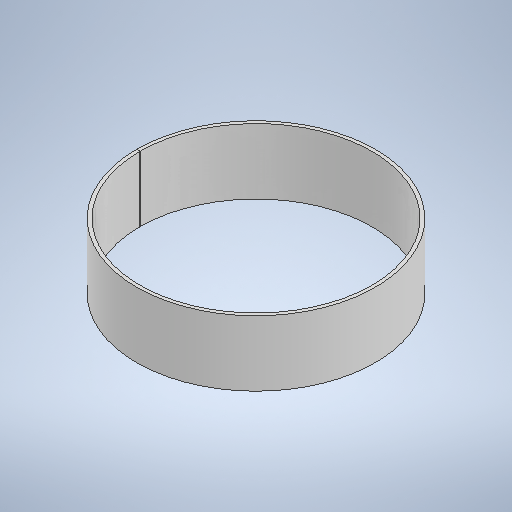
# Autodesk Inventor part: TZS 1204 accses hatch tube
Saved by Autodesk Inventor 2025 (Build 290162010, 162A)
## iProperties
Created: 2025-02-12
Part Number: TZS 1204 accses hatch tube
Material: Steel
Document SubType Name: Sheet Metal
Designer: pokla
Density: 7.85 g/cm^3
Flat Pattern Width: 11.6 cm
Flat Pattern Length: 131.056 cm
Flat Pattern Area: 1520.25 cm^2
Sheet Metal Rule: Default_mm
Sheet Metal Width: 116,000 mm
Sheet Metal Length: 1310,560 mm
Sheet Metal Area: 152024,918 mm^2
Appearance: Default
Mass: 13177.4 g
Surface Area: 5813.4 cm^2
Volume: 1678.65 cm^3
Author: pokla
Autodesk Inventor part; units mm, degrees
ref_plane "YZ Plane" through (0, 0, 0) normal (1, 0, 0) x (0, 1, 0)
ref_plane "XZ Plane" through (0, 0, 0) normal (0, 1, 0) x (-1, 0, 0)
ref_plane "XY Plane" through (0, 0, 0) normal (0, 0, 1) x (1, 0, 0)
sketch "Sketch1" plane through (0, 0, 0) normal (0, 1, 0) x (-1, 0, 0)
  line L0 (206, 66) -> (206, 0)
  line L1 (206, 0) -> (212, 0)
  line L2 (0, 0) -> (0, 109.131)
  line L3 (206, 66) -> (212, 66)
  line L4 (212, 0) -> (212, 66)
  line L5 (212, 0) -> (206, 0)
  line L6 (206, 0) -> (206, -50)
  line L7 (206, -50) -> (212, -50)
  line L8 (212, -50) -> (212, 0)
  point P0 (209, 0)
  point P1 (212, 0)
  point P2 (206, 0)
  point P3 (206, 0)
  dimension "d3" = 6
  dimension "d5" = 66
  dimension "d7" = 6
  dimension "d8" = 50
  dimension "d12" = 424
  constraints: 18 end point, 2 horizontal, 2 midpoint, 2 parallel, 2 perpendicular, 2 vertical, 1 horizontal alignment
  measures "d3" distance of L0.end L1.end
  measures "d5" distance between parallel lines of L1 L3
  measures "d7" distance of L6.end L7.end
  measures "d8" distance of L7.end L5.start
  measures "d12" diameter of L4 L2
revolve "Revolution1" add sketch "Sketch1" angle 359.9 about axis through (0, 0, 0) along (0, 0, 1)
sketch "Sketch2" plane through (0, 0, 0) normal (0, 1, 0) x (-1, 0, 0)
  circle A0 centre (0, -606) radius 606
  point P0 (0, 0)
  dimension "d9" = 1212
  constraints: 2 vertical alignment, 2 other
extrude "Extrusion1" [suppressed]
equation "\"d5\" = Accsess_hatch_lenght"
equation "\"d7\" = d3"
equation "\"BendRadius\" = Thickness"
equation "\"BendReliefWidth\" = Thickness"
equation "\"BendReliefDepth\" = 0.5 * Thickness"
equation "\"CornerReliefSize\" = 4 * Thickness"
equation "\"MinimumRemnant\" = 2 * Thickness"
equation "\"TransitionRadius\" = BendRadius"
equation "\"JacobiRadiusSize\" = BendRadius"
equation "\"GapSize\" = Thickness"
equation "\"Accsess_hatch_lenght\" = 66"
equation "\"Thickness\" = 6"
body "Solid1"
